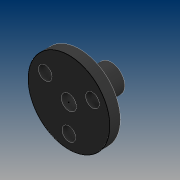
# Autodesk Inventor part: nakretka_na_igle
Saved by Autodesk Inventor 2021 (Build 250183000, 183)
## iProperties
Created: 2022-05-15
Part Number: nakretka_na_igle
Material: Generic
Document SubType Name: Modeling
Designer: agnpi
Density: 1 g/cm^3
Appearance: Rubber - Black
Author: agnpi
Autodesk Inventor part; units mm, degrees
ref_plane "YZ Plane" through (0, 0, 0) normal (1, 0, 0) x (0, 1, 0)
ref_plane "XZ Plane" through (0, 0, 0) normal (0, 1, 0) x (-1, 0, 0)
ref_plane "XY Plane" through (0, 0, 0) normal (0, 0, 1) x (1, 0, 0)
sketch "Sketch1" plane through (0, 0, 0) normal (0, 0, 1) x (1, 0, 0)
  line L0 (-13.3, 0) -> (13.3, 0) projected
  line L1 (0, -13.3) -> (0, 13.3) projected
  circle A0 centre (0, 0) radius 9.5
  circle A1 centre (0, 0) radius 1.3
  circle A2 centre (0, 0) radius 3.17
  dimension "d0" = 19
  dimension "d1" = 2.6
  dimension "d2" = 6.34
  constraints: 3 centre point, 3 coincident
  measures "d0" diameter of A0
  measures "d1" diameter of A1
  measures "d2" diameter of A2
extrude "Extrusion4" add sketch "Sketch1" along normal mid plane 2.5 contours A1 L1 A2 L0 | L0 A2 L1 A1 | A2 L1 A0 L0 | L0 A0 L1 A2 | A1 L0 A2 L1 | L1 A2 L0 A1 | A2 L0 A0 L1 | L1 A0 L0 A2
sketch "Sketch3" plane through (0, 0, -1.25) normal (0, 0, -1) x (-1, 0, 0)
  circle A0 centre (0, 0) radius 3.175
  circle A1 centre (0, 0) radius 1.3021
  dimension "d21" = 6.35
  constraints: 2 centre point, 2 coincident
  measures "d21" diameter of A0
extrude "Extrusion5" add sketch "Sketch3" along normal blind 7.36
sketch "Sketch4" plane through (0, 0, 1.25) normal (0, 0, 1) x (1, 0, 0)
  circle A0 centre (0, 0) radius 9.5 projected
  line L0 (-5.6994, 7.6005) -> (5.6994, 7.6005)
  arc A1 (5.6994, 7.6005) -> (-5.6994, 7.6005) centre (0, 0) ccw
  dimension "d27" = 11.3988
  constraints: 4 point on circle, 2 end point, 1 centre point, 1 concentric, 1 horizontal
  measures "d27" distance of L0.start L0.end
sketch "Sketch5" plane through (0, 0, 1.25) normal (0, 0, 1) x (1, 0, 0)
  point P0 (0, 0)
  point P1 (0, 0)
  constraints: 1 coincident
hole "Hole1" at (0, 0, 1.25) direction (0, 0, -1) diameter 3.5 end through all
sketch "Sketch6" plane through (0, 0, 1.25) normal (0, 0, 1) x (1, 0, 0)
  circle A0 centre (0, 0) radius 6.35 construction
  circle A1 centre (0, -6.35) radius 1.585
  line L0 (0, -13.3) -> (0, 13.3) construction
  line L1 (-13.3, 0) -> (13.3, 0) construction
  circle A2 centre (5.4993, 3.175) radius 1.585
  circle A3 centre (-5.4993, 3.175) radius 1.585
  dimension "d40" = 12.7
  dimension "d41" = 3.17
  dimension "d44" = 360
  constraints: 3 centre point, 1 coincident, 1 point on line, 1 vertical alignment, 9 other
  measures "d41" diameter of A1
extrude "Extrusion7" cut sketch "Sketch6" against normal through all
sketch "Sketch7" plane through (0, 0, 1.25) normal (0, 0, 1) x (1, 0, 0)
  circle A0 centre (0, 0) radius 9.5 projected
body "Solid4"
